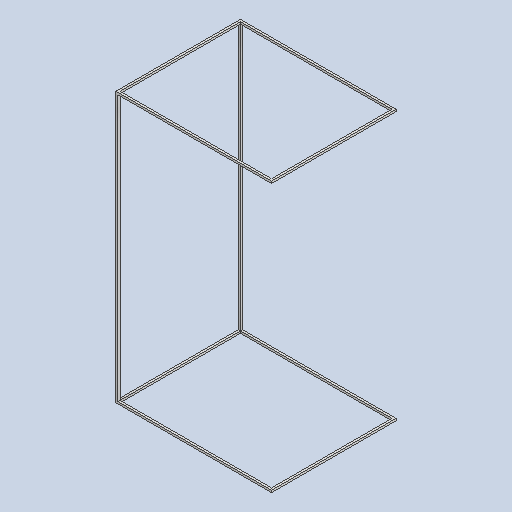
# Autodesk Inventor part: estrutura
Saved by Autodesk Inventor 2023 (Build 270158000, 158)
## iProperties
Created: 2022-08-29
Part Number: estrutura
Material: Generic
Document SubType Name: Modeling
Designer: cvss2
Density: 1 g/cm^3
Appearance: Default
Author: cvss2
Autodesk Inventor part; units mm, degrees
ref_plane "YZ Plane" through (0, 0, 0) normal (1, 0, 0) x (0, 1, 0)
ref_plane "XZ Plane" through (0, 0, 0) normal (0, 1, 0) x (-1, 0, 0)
ref_plane "XY Plane" through (0, 0, 0) normal (0, 0, 1) x (1, 0, 0)
sketch "Sketch1" plane through (0, 0, 0) normal (0, 0, 1) x (1, 0, 0)
  line L0 (0, 0) -> (1500, 0)
  line L1 (1500, 0) -> (1500, 2600)
  line L2 (1500, 2600) -> (0, 2600)
  line L3 (0, 2600) -> (0, 0)
  line L4 (0, 2600) -> (20, 2600)
  line L5 (20, 2600) -> (20, 2580)
  line L6 (20, 2580) -> (0, 2580)
  line L7 (0, 2580) -> (0, 2600)
  line L8 (1500, 2600) -> (1480, 2600)
  line L9 (1480, 2600) -> (1480, 2580)
  line L10 (1480, 2580) -> (1500, 2580)
  line L11 (1500, 2580) -> (1500, 2600)
  line L12 (1500, 0) -> (1480, 0)
  line L13 (1480, 0) -> (1480, 20)
  line L14 (1480, 20) -> (1500, 20)
  line L15 (1500, 20) -> (1500, 0)
  line L16 (0, 0) -> (20, 0)
  line L17 (20, 0) -> (20, 20)
  line L18 (20, 20) -> (0, 20)
  line L19 (0, 20) -> (0, 0)
  line L20 (20, 2580) -> (1480, 2580)
  line L21 (20, 2580) -> (20, 20)
  line L22 (20, 20) -> (1480, 20)
  line L23 (1480, 20) -> (1480, 2580)
  point P0 (1500, 2580)
  point P1 (1480, 2600)
  point P2 (1500, 20)
  point P3 (1480, 0)
  point P4 (0, 2580)
  point P5 (20, 2600)
  dimension "d0" = 1500
  dimension "d1" = 2600
  dimension "d2" = 20
  dimension "d3" = 20
  dimension "d4" = 20
  dimension "d5" = 20
  dimension "d6" = 20
  dimension "d7" = 20
  dimension "d8" = 20
  dimension "d9" = 20
  constraints: 48 end point, 10 parallel, 5 horizontal, 5 perpendicular
  measures "d0" distance of L2.end L1.end
  measures "d1" distance of L1.end L0.end
  measures "d2" distance of L5.end L6.end
  measures "d3" distance of L4.end L5.end
  measures "d4" distance of L10.end L9.end
  measures "d5" distance of L9.end L8.end
  measures "d6" distance of L13.end L14.end
  measures "d7" distance of L12.end L13.end
  measures "d8" distance of L18.end L17.end
  measures "d9" distance from line of L16.end L18
extrude "Extrusion1" add sketch "Sketch1" along normal blind 1200 contours L3 L18 L17 L0 | L13 L14 L1 L0 | L3 L2 L5 L6 | L9 L2 L1 L10
extrude "Extrusion2" add sketch "Sketch1" along normal blind 20 contours L17 L22 L13 L0 | L3 L6 L21 L18 | L5 L2 L9 L20
sketch "Sketch2" plane through (0, 0, 1200) normal (0, 0, 1) x (1, 0, 0)
  line L0 (0, 20) -> (0, 0) projected
  line L1 (0, 0) -> (20, 0) projected
  line L2 (20, 0) -> (20, 20) projected
  line L3 (20, 20) -> (0, 20) projected
  line L4 (20, 2580) -> (20, 2600) projected
  line L5 (20, 2600) -> (0, 2600) projected
  line L6 (0, 2600) -> (0, 2580) projected
  line L7 (0, 2580) -> (20, 2580) projected
  line L8 (1480, 20) -> (1480, 0) projected
  line L9 (1480, 0) -> (1500, 0) projected
  line L10 (1500, 0) -> (1500, 20) projected
  line L11 (1500, 20) -> (1480, 20) projected
  line L12 (1500, 2580) -> (1500, 2600) projected
  line L13 (1500, 2600) -> (1480, 2600) projected
  line L14 (1480, 2600) -> (1480, 2580) projected
  line L15 (1480, 2580) -> (1500, 2580) projected
  line L16 (20, 0) -> (20, 20) projected
  line L17 (1480, 20) -> (1480, 0) projected
  line L18 (1480, 20) -> (20, 20)
  line L19 (1480, 2600) -> (1480, 2580) projected
  line L20 (1480, 2600) -> (20, 2600) projected
  line L21 (20, 2580) -> (20, 2600) projected
  line L22 (20, 2580) -> (1480, 2580) projected
  line L23 (1480, 20) -> (20, 20) projected
  line L24 (20, 2580) -> (1480, 2580) projected
  line L25 (0, 2580) -> (20, 2580) projected
  line L26 (0, 2580) -> (0, 20) projected
  line L27 (20, 20) -> (0, 20) projected
  line L28 (20, 20) -> (20, 2580) projected
  line L29 (20, 0) -> (20, 20) projected
  line L30 (1480, 20) -> (1480, 0) projected
  line L31 (1480, 2600) -> (1480, 2580) projected
  line L32 (1480, 2600) -> (20, 2600) projected
  line L33 (20, 2580) -> (20, 2600) projected
  line L34 (20, 0) -> (1480, 0)
  line L35 (0, 0) -> (1500, 0) projected
  constraints: 4 end point, 1 horizontal, 1 other
extrude "Extrusion3" add sketch "Sketch2" against normal blind 20 contours L26 L7 L28 L3 | L18 L8 L34 L2 | L4 L20 L14 L22
equation "\"d0\" = comprimento"
equation "\"d1\" = largura"
equation "\"comprimento\" = 1500"
equation "\"largura\" = 2600"
body "Solid1"
